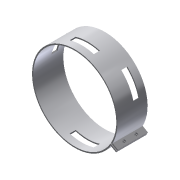
# Autodesk Inventor part: ring
Saved by Autodesk Inventor 2015 (Build 190159000, 159)
## iProperties
Created: 2015-10-29
Part Number: ring
Material: Generic
Document SubType Name: Modeling
Designer: jad211
Density: 1 g/cm^3
Appearance: Default
Author: jad211
Autodesk Inventor part; units mm, degrees
sketch "Sketch1" plane through (0, 0, 0) normal (0, 1, 0) x (-1, 0, 0)
  circle A0 centre (0, 0) radius 34.5
  circle A1 centre (0, 0) radius 35.5
  dimension "d0" = 69
  dimension "d1" = 71
  constraints: 2 centre point, 2 coincident
  measures "d0" diameter of A0
  measures "d1" diameter of A1
extrude "Extrusion1" add sketch "Sketch1" along normal blind 25
ref_plane "Work Plane1" through (0, 0, 35.5) normal (0, 0, 1) x (1, 0, 0)
ref_plane "Work Plane2" through (0, 0, -35.5) normal (0, 0, 1) x (1, 0, 0)
ref_plane "Work Plane3" through (0, 0, 0) normal (0.866, 0, -0.5) x (0, 1, 0)
ref_plane "Work Plane6" through (30.7439, 0, 17.75) normal (0.866, 0, 0.5) x (0, 1, 0)
ref_plane "Work Plane5" through (0, 0, 0) normal (0.866, 0, 0.5) x (0, 1, 0)
sketch "Sketch3" plane through (0, 0, 35.5) normal (0, 0, 1) x (1, 0, 0)
  line L0 (-10, 10.828) -> (10, 10.828)
  line L1 (10, 10.828) -> (10, 5.828)
  line L2 (10, 5.828) -> (-10, 5.828)
  line L3 (-10, 5.828) -> (-10, 10.828)
  line L4 (-35.5, 0) -> (35.5, 0) projected
  point P0 (0, 0)
  dimension "d6" = 10.828
  dimension "d7" = 5
  dimension "d8" = 10
  dimension "d9" = 20
  constraints: 8 end point, 2 parallel, 1 horizontal, 1 perpendicular
  measures "d6" distance between parallel lines of L0 L4
  measures "d7" distance of L2.end L0.start
  measures "d8" distance from line of point (0, 0) L3
  measures "d9" distance between parallel lines of L3 L1
sketch "Sketch4" plane through (0, 0, -35.5) normal (0, 0, 1) x (1, 0, 0)
  line L0 (-10, 5.828) -> (10, 5.828)
  line L1 (10, 5.828) -> (10, 10.828)
  line L2 (10, 10.828) -> (-10, 10.828)
  line L3 (-10, 10.828) -> (-10, 5.828)
  point P0 (0, 0)
  dimension "d10" = 10.828
  dimension "d11" = 5
  dimension "d12" = 10
  dimension "d13" = 20
  constraints: 8 end point, 2 parallel, 1 horizontal, 1 perpendicular
  measures "d10" distance from line of point (0, 0) L2
  measures "d11" distance of L2.end L0.start
  measures "d12" distance from line of point (0, 0) L3
  measures "d13" distance between parallel lines of L3 L1
ref_plane "Work Plane7" through (-30.7439, 0, 17.75) normal (0.866, 0, -0.5) x (0, 1, 0)
sketch "Sketch5" plane through (-30.7439, 0, 17.75) normal (0.866, 0, -0.5) x (0, 1, 0)
  line L0 (19.172, 10) -> (14.172, 10)
  line L1 (14.172, 10) -> (14.172, -10)
  line L2 (14.172, -10) -> (19.172, -10)
  line L3 (19.172, -10) -> (19.172, 10)
  line L4 (25, -35.5) -> (25, 35.5) projected
  point P0 (0, 0)
  dimension "d14" = 10.828
  dimension "d15" = 5
  dimension "d16" = 10
  dimension "d17" = 20
  constraints: 8 end point, 2 parallel, 1 horizontal, 1 perpendicular
  measures "d14" distance between parallel lines of L4 L1
  measures "d15" distance of L0.start L0.end
  measures "d16" distance from line of point (0, 0) L0
  measures "d17" distance between parallel lines of L0 L2
sketch "Sketch6" plane through (30.7439, 0, 17.75) normal (0.866, 0, 0.5) x (0, 1, 0)
  line L0 (14.172, 10) -> (19.172, 10)
  line L1 (19.172, 10) -> (19.172, -10)
  line L2 (19.172, -10) -> (14.172, -10)
  line L3 (14.172, -10) -> (14.172, 10)
  line L4 (25, -35.5) -> (25, 35.5) projected
  point P0 (0, 0)
  dimension "d18" = 10.828
  dimension "d19" = 5
  dimension "d20" = 20
  dimension "d21" = 10
  constraints: 8 end point, 2 parallel, 1 horizontal, 1 perpendicular
  measures "d18" distance between parallel lines of L4 L3
  measures "d19" distance of L1.end L2.end
  measures "d20" distance between parallel lines of L2 L0
  measures "d21" distance from line of point (0, 0) L0
extrude "Extrusion2" cut sketch "Sketch3" against normal blind 25
extrude "Extrusion3" cut sketch "Sketch6" against normal blind 25
extrude "Extrusion4" cut sketch "Sketch4" along normal blind 25
extrude "Extrusion5" cut sketch "Sketch5" along normal blind 25
ref_plane "Work Plane8" through (30.7439, 0, -17.75) normal (0.866, 0, -0.5) x (0, 1, 0)
sketch "Sketch7" plane through (30.7439, 0, -17.75) normal (0.866, 0, -0.5) x (0, 1, 0)
  line L0 (25, -0.5) -> (0, -0.5)
  line L1 (0, -0.5) -> (0, 0.5)
  line L2 (0, 0.5) -> (25, 0.5)
  line L3 (25, 0.5) -> (25, -0.5)
  line L4 (25, -0.5) -> (0, 0.5) construction
  line L5 (0, -0.5) -> (25, 0.5) construction
  point P0 (0, 0)
  point P1 (12.5, 0)
  dimension "d30" = 25
  dimension "d31" = 1
  dimension "d32" = 0.5
  constraints: 12 end point, 2 midpoint, 2 parallel, 1 horizontal, 1 perpendicular
  measures "d30" distance between parallel lines of L3 L1
  measures "d31" distance of L0.end L1.end
  measures "d32" distance from line of point (0, 0) L2
extrude "Extrusion6" cut sketch "Sketch7" against normal blind 25
sketch "Sketch8" plane through (30.7439, 0, -17.75) normal (0.866, 0, -0.5) x (0, 1, 0)
  line L0 (25, 34.5) -> (25, -34.5) projected
  line L1 (0, 0.5) -> (25, 0.5)
  line L2 (25, 0.5) -> (25, 1.5)
  line L3 (25, 1.5) -> (0, 1.5)
  line L4 (0, 1.5) -> (0, 0.5)
  line L5 (0, -0.5) -> (25, -0.5)
  line L6 (25, -0.5) -> (25, -1.5)
  line L7 (25, -1.5) -> (0, -1.5)
  line L8 (0, -1.5) -> (0, -0.5)
  point P0 (0, 0)
  point P1 (25, 0.5)
  dimension "d35" = 1
  dimension "d36" = 1
  constraints: 16 end point, 4 parallel, 2 horizontal, 2 perpendicular, 2 point on line
  measures "d35" distance between parallel lines of L1 L3
  measures "d36" distance between parallel lines of L5 L7
extrude "Extrusion7" add sketch "Sketch8" along normal blind 5
sketch "Sketch9" plane through (31.4939, 0, -16.451) normal (0.5, 0, 0.866) x (0.866, 0, -0.5)
  circle A0 centre (2.5, 7.5) radius 1.25
  circle A1 centre (2.5, 17.5) radius 1.25
  line L0 (0, 0) -> (5, 0) projected
  line L1 (0, 25) -> (5, 25) projected
  line L2 (5, 25) -> (5, 0) projected
  point P0 (-35.5, 0)
  dimension "d39" = 2.5
  dimension "d40" = 2.5
  dimension "d44" = 2.5
  dimension "d45" = 2.5
  dimension "d46" = 7.5
  dimension "d47" = 7.5
  constraints: 2 centre point
  measures "d39" diameter of A0
  measures "d40" diameter of A1
  measures "d44" distance from line of L2 A1.centre
  measures "d45" distance from line of L2 A0.centre
  measures "d46" distance from line of L0 A0.centre
  measures "d47" distance from line of L1 A1.centre
extrude "Extrusion8" cut sketch "Sketch9" against normal blind 5
equation "\"d9\" = 2 * d8"
equation "\"d10\" = d6"
equation "\"d12\" = d8"
equation "\"d13\" = 2 * d12"
equation "\"d14\" = d6"
equation "\"d15\" = d7"
equation "\"d17\" = 2 * d16"
equation "\"d18\" = d6"
equation "\"d19\" = d7"
equation "\"d20\" = d17"
equation "\"d21\" = d8"
equation "\"d32\" = 0.5 * d31"
body "Solid1"
